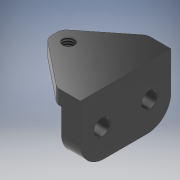
# Autodesk Inventor part: X-Axis_Z_Endstop_Bracket_LM3047
Saved by Autodesk Inventor 2020.3 (Build 243373000, 373)
## iProperties
Created: 2020-06-09
Part Number: X-Axis_Z_Endstop_Bracket_LM3047
Material: ABS Plastic
Document SubType Name: Modeling
Designer: rah75
Density: 1.06 g/cm^3
Appearance: Satin - Black
Author: rah75
Autodesk Inventor part; units mm, degrees
ref_plane "YZ Plane" through (0, 0, 0) normal (1, 0, 0) x (0, 1, 0)
ref_plane "XZ Plane" through (0, 0, 0) normal (0, 1, 0) x (-1, 0, 0)
ref_plane "XY Plane" through (0, 0, 0) normal (0, 0, 1) x (1, 0, 0)
sketch "Sketch1" plane through (0, 0, 0) normal (0, 0, 1) x (1, 0, 0)
  line L0 (-4, -13) -> (0, -13)
  line L1 (0, -13) -> (0, 0)
  line L2 (0, 0) -> (-15, 0)
  line L3 (-15, 0) -> (-15, -3)
  line L4 (-15, -3) -> (-4, -3)
  line L5 (-4, -3) -> (-4, -13)
  dimension "d0" = 3
  dimension "d1" = 4
  dimension "d2" = 10
  dimension "d3" = 15
  constraints: 12 end point, 5 perpendicular, 1 coincident, 1 horizontal
  measures "d0" distance of L2.end L3.end
  measures "d1" distance of L0.start L0.end
  measures "d2" distance of L4.end L0.start
  measures "d3" distance of L1.end L2.end
extrude "Extrusion1" add sketch "Sketch1" along normal mid plane 19.05
sketch "Sketch2" plane through (-4, -13, 9.525) normal (-1, 0, 0) x (0, 0, 1)
  line L0 (-19.05, 0) -> (0, 0) projected
  line L1 (0, 10) -> (0, 0) projected
  line L2 (-19.05, 10) -> (0, 10) projected
  line L3 (-19.05, 0) -> (-19.05, 10) projected
  line L4 (-19.05, 0) -> (-19.05, 10) projected
  line L5 (-19.05, 13) -> (0, 13) projected
  line L6 (-19.05, 0) -> (0, 0) projected
  point P0 (-9.525, 13)
  point P1 (-14.525, 6)
  point P2 (-4.525, 6)
  point P3 (-19.05, 5)
  point P4 (-9.525, 13)
  point P5 (-9.525, 0)
  dimension "d6" = 10
  dimension "d31" = 7
  dimension "d32" = 5
  constraints: 3 midpoint, 1 horizontal alignment
  measures "d6" distance of point (-4.525, 6) point (-14.525, 6)
  measures "d31" distance from line of point (-4.525, 6) L5
  measures "d32" horizontal distance of point (-9.525, 0) point (-14.525, 6)
hole "Hole1" at (-4, -7, -5) at (-4, -7, 5) direction (1, 0, 0) diameter 3.4 depth 8.7884 clearance for "Socket Head Cap Screw" size "M3" standard "Ansi Metric M Profile"
sketch "Sketch3" plane through (-15, 0, 9.525) normal (0, 1, 0) x (1, 0, 0)
  line L0 (15, 19.05) -> (15, 0) projected
  point P0 (15, 9.525)
  point P1 (3, 9.525)
  point P2 (15, 9.525)
  dimension "d15" = 12
  constraints: 1 horizontal alignment, 1 midpoint
  measures "d15" distance from line of point (3, 9.525) L0
hole "Hole2" at (-12, 0, 0) direction (0, -1, 0) diameter 2.459 depth 8.8 thread size "M3x0.5" class "6H" standard "ANSI Metric M Profile"
chamfer "Chamfer1" distance 10 distance2 8 1 edges at (-15, -1.5, 9.525) measured on face at (-1.3333, -5.3333, 9.525)
chamfer "Chamfer2" distance 10 distance2 8 1 edges at (-15, -1.5, -9.525) measured on face at (-1.3333, -5.3333, -9.525)
fillet "Fillet1" radius 2 4 edges at (-5, -1.5, -9.525) (-15, -1.5, -1.525) (-15, -1.5, 1.525) (-5, -1.5, 9.525)
fillet "Fillet1" radius 5 2 edges at (-2, -13, -9.525) (-2, -13, 9.525)
body "Solid1"
